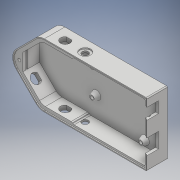
# Autodesk Inventor part: Arduino simple 4 channel ttl bottom
Saved by Autodesk Inventor 2017 (Build 210142000, 142)
## iProperties
Created: 2016-10-03
Part Number: Arduino simple 4 channel ttl bottom
Material: Generic
Document SubType Name: Modeling
Designer: andrew
Density: 1 g/cm^3
Appearance: Default
Author: andrew
Autodesk Inventor part; units mm, degrees
ref_plane "YZ Plane" through (0, 0, 0) normal (1, 0, 0) x (0, 1, 0)
ref_plane "XZ Plane" through (0, 0, 0) normal (0, 1, 0) x (-1, 0, 0)
ref_plane "XY Plane" through (0, 0, 0) normal (0, 0, 1) x (1, 0, 0)
sketch "Sketch1" plane through (0, 0, 0) normal (0, 1, 0) x (-1, 0, 0)
  circle A0 centre (66.1, -35.5) radius 2.345
  circle A1 centre (15.3, -50.7) radius 2.345
  circle A2 centre (14, -2.5) radius 2.345
  circle A3 centre (66.1, -7.6) radius 2.345
  line L0 (0, 0) -> (68.6, 0) construction
  line L1 (0, -53.3) -> (0, 0) construction
  line L2 (66.1, -53.3) -> (0, -53.3) construction
  line L3 (66.1, -40.6) -> (66.1, -53.3) construction
  line L4 (68.6, -40.6) -> (66.1, -40.6) construction
  line L5 (68.6, 0) -> (68.6, -40.6) construction
  line L6 (0, -12.2) -> (0, -3.3) construction
  line L7 (-1.8, -3.3) -> (0, -3.3) construction
  line L8 (-1.8, -12.2) -> (-1.8, -3.3) construction
  line L9 (0, -12.2) -> (-1.8, -12.2) construction
  line L10 (-6.2, -43.5895) -> (-6.2, -31.5895) construction
  line L11 (0, -43.5895) -> (0, -31.5895) construction
  line L12 (-6.2, -31.5895) -> (0, -31.5895) construction
  line L13 (-6.2, -43.5895) -> (-6.2, -31.5895) construction
  line L14 (0, -43.5895) -> (-6.2, -43.5895) construction
  circle A4 centre (14, -2.5) radius 1.6
  circle A5 centre (15.3, -50.7) radius 1.6
  circle A6 centre (66.1, -35.5) radius 1.6
  circle A7 centre (66.1, -7.6) radius 1.6
  constraints: 30 end point, 8 centre point
extrude "Extrusion1" add sketch "Sketch1" along normal blind 4.69
draft "FaceDraft1" angle 25 pull direction (0, -1, 0) faces at (-68.4146, 3.1267, -7.9762) (-64.2253, 3.1267, -36.9087) (-16.3146, 3.1267, -2.8762) (-17.6146, 3.1267, -51.0762) fixed edges at (-63.755, 0, -7.6) (-63.755, 0, -35.5) (-11.655, 0, -2.5) (-12.955, 0, -50.7)
sketch "Sketch2" plane through (-66.1, 4.69, -7.6) normal (0, 1, 0) x (1, 0, 0)
  circle A0 centre (0.0002, 27.8999) radius 2.345 construction
  circle A1 centre (50.8002, 43.0999) radius 2.345 construction
  circle A2 centre (52.1002, -5.1001) radius 2.345 construction
  circle A3 centre (0.0002, -0.0001) radius 2.345 construction
  line L0 (66.1002, -7.6001) -> (-2.4998, -7.6001) construction
  line L1 (66.1002, 45.6999) -> (66.1002, -7.6001) construction
  line L2 (0.0002, 45.6999) -> (66.1002, 45.6999) construction
  line L3 (0.0002, 32.9999) -> (0.0002, 45.6999) construction
  line L4 (-2.4998, 32.9999) -> (0.0002, 32.9999) construction
  line L5 (-2.4998, -7.6001) -> (-2.4998, 32.9999) construction
  line L6 (66.1002, 4.5999) -> (66.1002, -4.3001) construction
  line L7 (67.9002, -4.3001) -> (66.1002, -4.3001) construction
  line L8 (66.1002, 4.5999) -> (67.9002, 4.5999) construction
  line L9 (72.3002, 35.9894) -> (72.3002, 23.9894) construction
  line L10 (66.1002, 35.9894) -> (66.1002, 23.9894) construction
  line L11 (72.3002, 23.9894) -> (66.1002, 23.9894) construction
  line L12 (72.3002, 35.9894) -> (72.3002, 23.9894) construction
  line L13 (66.1002, 35.9894) -> (72.3002, 35.9894) construction
  circle A4 centre (52.1002, -5.1001) radius 1.6 construction
  circle A5 centre (50.8002, 43.0999) radius 1.6 construction
  circle A6 centre (0.0002, 27.8999) radius 1.6 construction
  circle A7 centre (0.0002, -0.0001) radius 1.6 construction
  line L14 (-4.4998, -9.6001) -> (68.1002, -9.6001) construction
  line L15 (-1.9998, 47.6999) -> (-1.9998, 34.9999) construction
  line L16 (-1.9998, 34.9999) -> (-4.4998, 34.9999) construction
  line L17 (66.1002, 4.5999) -> (74.6809, 4.5999) construction
  line L18 (74.6809, 4.5999) -> (74.6809, -4.3001) construction
  line L19 (74.6809, -4.3001) -> (66.1002, -4.3001) construction
  line L20 (66.1002, -4.3001) -> (66.1002, 4.5999) construction
  line L21 (66.1002, 23.9894) -> (80.0982, 23.9894) construction
  line L22 (80.0982, 23.9894) -> (80.0982, 35.9894) construction
  line L23 (80.0982, 35.9894) -> (66.1002, 35.9894) construction
  line L24 (66.1002, 35.9894) -> (66.1002, 23.9894) construction
  line L25 (76.0853, 6.0043) -> (64.6958, 6.0043) construction
  line L26 (64.6958, 6.0043) -> (64.6958, -5.7045) construction
  line L27 (64.6958, -5.7045) -> (76.0853, -5.7045) construction
  line L28 (76.0853, -5.7045) -> (76.0853, 6.0043) construction
  line L29 (82.0982, 21.9894) -> (64.1002, 21.9894) construction
  line L30 (64.1002, 21.9894) -> (64.1002, 37.9894) construction
  line L31 (64.1002, 37.9894) -> (82.0982, 37.9894) construction
  line L32 (82.0982, 37.9894) -> (82.0982, 21.9894) construction
  line L33 (68.1002, 6.0043) -> (71.1002, 6.0043)
  line L34 (71.1002, 21.9894) -> (68.1002, 21.9894)
  line L35 (71.1002, 37.9894) -> (68.1002, 37.9894)
  line L36 (68.1002, -5.7045) -> (68.1002, -9.6001)
  line L37 (68.1002, -9.6001) -> (68.1002, -4.3001) construction
  line L38 (68.1002, 6.0043) -> (68.1002, 47.6999) construction
  line L39 (68.1002, 47.6999) -> (68.1002, 37.9894)
  line L40 (68.1002, 21.9894) -> (68.1002, 6.0043)
  line L41 (71.1002, 37.9894) -> (71.1002, 50.6999)
  line L42 (68.1002, -9.6001) -> (68.1002, -11.1001)
  line L43 (68.1002, 47.6999) -> (68.1002, 49.1999)
  line L44 (68.1002, 47.6999) -> (69.6002, 47.6999) construction
  line L45 (71.1002, 50.6999) -> (71.1002, 52.1999)
  line L46 (71.1002, 50.6999) -> (72.6002, 50.6999) construction
  line L47 (68.1002, 49.1999) -> (-6.7498, 49.1999)
  line L48 (68.1002, -11.1001) -> (-6.7498, -11.1001)
  line L49 (71.1002, -14.1001) -> (71.1002, -5.7045)
  line L50 (71.1002, 6.0043) -> (71.1002, 21.9894)
  line L51 (71.1002, -5.7045) -> (68.1002, -5.7045)
  line L52 (-15.2028, 65.0749) -> (-15.2028, 33.3249) construction
  line L53 (-16.7928, 49.1999) -> (-16.7928, 33.3249) construction
  line L54 (-21.7478, 49.1999) -> (-16.7928, 49.1999) construction
  line L55 (-21.7478, 33.3249) -> (-21.7478, 65.0749) construction
  line L56 (-15.2028, 33.3249) -> (-28.2928, 33.3249) construction
  line L57 (-15.2028, 49.1999) -> (-28.2928, 49.1999) construction
  line L58 (-35.9958, 47.6999) -> (-8.2498, 47.6999)
  line L59 (-16.7928, 33.3249) -> (-26.7028, 33.3249) construction
  line L60 (-53.1418, 1.9038) -> (-56.6456, 5.4076) construction
  line L61 (-56.6456, 5.4076) -> (-45.4202, 16.6329) construction
  line L62 (-45.4202, 16.6329) -> (-38.4128, 9.6254) construction
  line L63 (-46.5445, 17.7572) -> (-37.2885, 8.5011) construction
  line L64 (-68.9952, -4.6935) -> (-46.5445, 17.7572) construction
  line L65 (-57.7699, 6.5319) -> (-48.5138, -2.7242) construction
  line L66 (-38.4128, 9.6254) -> (-49.6381, -1.5999) construction
  line L67 (-42.0062, -7.1105) -> (-62.1562, 13.0395)
  line L68 (-41.9165, 13.1292) -> (-64.3672, -9.3215) construction
  line L69 (-45.1882, -10.2925) -> (-65.3382, 9.8575)
  line L70 (-37.2885, 8.5011) -> (-59.7391, -13.9495) construction
  line L71 (-59.7391, -13.9495) -> (-68.9952, -4.6935) construction
  arc A8 (-65.3382, 28.2423) -> (-65.3382, 9.8575) centre (-56.1458, 19.0499) ccw
  arc A9 (-62.1562, 25.0603) -> (-62.1562, 13.0395) centre (-56.1458, 19.0499) ccw
  line L72 (-8.2498, -9.6001) -> (-35.9958, -9.6001)
  arc A10 (-42.0062, -7.1105) -> (-35.9958, -9.6001) centre (-35.9958, -1.1001) ccw
  arc A11 (-45.1882, -10.2925) -> (-35.9958, -14.1001) centre (-35.9958, -1.1001) ccw
  line L73 (-28.2928, 33.3249) -> (-28.2928, 65.0749) construction
  line L74 (-26.7028, 33.3249) -> (-26.7028, 49.1999) construction
  arc A12 (-35.9958, 47.6999) -> (-42.0062, 45.2103) centre (-35.9958, 39.1999) ccw
  arc A13 (-35.9958, 52.1999) -> (-45.1882, 48.3923) centre (-35.9958, 39.1999) ccw
  line L75 (-65.3382, 28.2423) -> (-45.1882, 48.3923)
  line L76 (-62.1562, 25.0603) -> (-42.0062, 45.2103)
  line L77 (-7.4998, -10.3501) -> (-7.4998, -10.3501)
  line L78 (-7.4998, 48.4499) -> (-7.4998, 48.4499)
  line L79 (-35.9958, -14.1001) -> (71.1002, -14.1001)
  line L80 (-35.9958, 52.1999) -> (71.1002, 52.1999)
  line L81 (-8.2498, -9.6001) -> (-6.7498, -11.1001)
  line L82 (-8.2498, 47.6999) -> (-6.7498, 49.1999)
  line L83 (-52.0812, 2.9645) -> (-59.329, 10.2123) construction
  line L84 (-59.329, 10.2123) -> (-59.329, 27.8875) construction
  point P0 (66.1, -7.6)
  point P1 (66.1002, -7.6001)
  point P2 (-40.1379, -11.1001)
  point P3 (-70.2879, 19.0499)
  dimension "d7" = 2
  dimension "d9" = 2
  dimension "d51" = 1.5
  dimension "d53" = 1.5
  dimension "d54" = 90
  dimension "d55" = 1.5
  dimension "d56" = 90
  dimension "d146" = 4.955
  dimension "d147" = 9.91
  dimension "d152" = 31.75
  dimension "d153" = 13.09
  dimension "d154" = 4.955
  dimension "d155" = 9.91
  dimension "d204" = 10.25
  dimension "d205" = 17.6751
  constraints: 170 end point, 20 point on line, 14 centre point, 13 perpendicular, 12 point on circle, 11 parallel, 10 midpoint, 8 horizontal, 5 vertical, 1 coincident, 1 collinear, 11 other
  measures "d7" distance between parallel lines of L0 L14
  measures "d9" distance between parallel lines of L21 L29
  measures "d51" distance of L14.end L42.end
  measures "d53" distance of L38.end L43.end
  measures "d54" angle of L44 L43
  measures "d55" distance of L41.end L45.end
  measures "d56" angle of L46 L45
  measures "d146" distance of L60.start L60.end
  measures "d147" distance of L62.start L66.start
  measures "d152" distance of L56.end L73.end
  measures "d153" distance of L56.start L56.end
  measures "d154" distance of L54.start L53.start
  measures "d155" distance of L59.start L74.start
  measures "d204" distance of L83.start L83.end
  measures "d205" distance of L83.end L84.end
extrude "Extrusion2" add sketch "Sketch2" against normal blind 17.29
sketch "Sketch4" plane through (-66.1, -12.6, -7.6) normal (0, -1, 0) x (1, 0, 0)
  line L0 (-85.6267, 83.4161) -> (-53.8767, 83.4161)
  line L1 (-53.8767, 83.4161) -> (-53.8767, 70.3261)
  line L2 (-53.8767, 70.3261) -> (-85.6267, 70.3261)
  line L3 (-85.6267, 70.3261) -> (-85.6267, 83.4161)
  line L4 (-53.8767, 76.8711) -> (-85.6267, 76.8711)
  line L5 (-69.7517, 83.4161) -> (-69.7517, 70.3261)
  line L6 (-69.7517, 76.8711) -> (-69.7517, 81.8261)
  line L7 (-69.7517, 81.8261) -> (-53.8767, 81.8261)
  line L8 (-53.8767, 81.8261) -> (-53.8767, 71.9161)
  line L9 (-53.8767, 71.9161) -> (-69.7517, 71.9161)
  line L10 (-85.7515, 30.5625) -> (-63.3008, 53.0132)
  line L11 (-63.3008, 53.0132) -> (-54.0448, 43.7571)
  line L12 (-54.0448, 43.7571) -> (-76.4954, 21.3065)
  line L13 (-76.4954, 21.3065) -> (-85.7515, 30.5625)
  line L14 (-58.6728, 48.3851) -> (-81.1234, 25.9345)
  line L15 (-74.5261, 41.7878) -> (-65.2701, 32.5318)
  line L16 (-69.8981, 37.1598) -> (-73.4018, 40.6635)
  line L17 (-73.4018, 40.6635) -> (-62.1765, 51.8889)
  line L18 (-62.1765, 51.8889) -> (-55.1691, 44.8814)
  line L19 (-55.1691, 44.8814) -> (-66.3944, 33.6561)
  line L20 (-56.2658, 116.7338) -> (-33.8151, 94.2832)
  line L21 (-33.8151, 94.2832) -> (-43.0711, 85.0271)
  line L22 (-43.0711, 85.0271) -> (-65.5218, 107.4778)
  line L23 (-65.5218, 107.4778) -> (-56.2658, 116.7338)
  line L24 (-38.4431, 89.6551) -> (-60.8938, 112.1058)
  line L25 (-45.0404, 105.5085) -> (-54.2965, 96.2524)
  line L26 (-49.6685, 100.8805) -> (-46.1647, 104.3842)
  line L27 (-46.1647, 104.3842) -> (-34.9394, 93.1589)
  line L28 (-34.9394, 93.1589) -> (-41.9468, 86.1514)
  line L29 (-41.9468, 86.1514) -> (-53.1722, 97.3767)
  line L30 (71.1002, -52.1999) -> (-7.4998, -52.1999)
  line L31 (-7.4998, -52.1999) -> (-7.4998, 14.1001)
  line L32 (-7.4998, 14.1001) -> (71.1002, 14.1001)
  line L33 (71.1002, 14.1001) -> (71.1002, -52.1999)
  line L34 (68.1002, 11.1001) -> (68.1002, 5.7045) projected
  line L35 (68.1002, -49.1999) -> (-6.7498, -49.1999) projected
  line L36 (68.1002, 11.1001) -> (-4.4998, 11.1001)
  line L37 (-4.4998, 11.1001) -> (-4.4998, -49.1999)
  line L38 (-4.4998, -49.1999) -> (68.1002, -49.1999)
  line L39 (68.1002, -49.1999) -> (68.1002, 11.1001)
  line L40 (-4.4998, -49.1999) -> (34.0716, -49.1999) construction
  line L41 (-7.4998, 14.1001) -> (-7.4998, -52.1999) projected
  line L42 (-7.4998, -19.0499) -> (35.1392, -19.0499) construction
  line L43 (-38.4431, -92.3206) -> (-68.5931, -122.4706)
  line L44 (-38.4431, -152.6206) -> (-68.5931, -122.4706)
  line L45 (-69.3715, -144.1429) -> (-46.9208, -121.6922)
  line L46 (-46.9208, -121.6922) -> (-37.6648, -130.9483)
  line L47 (-37.6648, -130.9483) -> (-60.1154, -153.3989)
  line L48 (-38.7891, -129.824) -> (-50.0144, -141.0493)
  line L49 (-45.7965, -122.8165) -> (-38.7891, -129.824)
  line L50 (-57.0218, -134.0419) -> (-45.7965, -122.8165)
  line L51 (-53.5181, -137.5456) -> (-57.0218, -134.0419)
  line L52 (-58.1461, -132.9176) -> (-48.8901, -142.1736)
  line L53 (-60.1154, -153.3989) -> (-69.3715, -144.1429)
  line L54 (-42.2928, -126.3203) -> (-64.7435, -148.7709)
  line L55 (-37.6648, -113.9929) -> (-46.9208, -123.2489)
  line L56 (-38.7891, -115.1172) -> (-45.7965, -122.1246)
  line L57 (-45.7965, -122.1246) -> (-57.0218, -110.8993)
  line L58 (-50.0144, -103.8919) -> (-38.7891, -115.1172)
  line L59 (-48.8901, -102.7676) -> (-58.1461, -112.0236)
  line L60 (-46.9208, -123.2489) -> (-69.3715, -100.7983)
  line L61 (-42.2928, -118.6209) -> (-64.7435, -96.1703)
  line L62 (-60.1154, -91.5422) -> (-37.6648, -113.9929)
  line L63 (-69.3715, -100.7983) -> (-60.1154, -91.5422)
  line L64 (-53.5181, -107.3956) -> (-50.0144, -103.8919)
  line L65 (58.0279, 196.0229) -> (58.0279, 164.2729)
  line L66 (58.0279, 164.2729) -> (44.9379, 164.2729)
  line L67 (44.9379, 164.2729) -> (44.9379, 196.0229)
  line L68 (44.9379, 196.0229) -> (58.0279, 196.0229)
  line L69 (51.4829, 164.2729) -> (51.4829, 196.0229)
  line L70 (58.0279, 180.1479) -> (44.9379, 180.1479)
  line L71 (51.4829, 180.1479) -> (56.4379, 180.1479)
  line L72 (56.4379, 180.1479) -> (56.4379, 164.2729)
  line L73 (56.4379, 164.2729) -> (46.5279, 164.2729)
  line L74 (46.5279, 164.2729) -> (46.5279, 180.1479)
  line L75 (-7.4998, 14.1001) -> (-7.4998, -52.1999)
  line L76 (-68.9952, -42.7933) -> (-46.5445, -20.3426) construction
  line L77 (-46.5445, -20.3426) -> (-37.2885, -29.5987) construction
  line L78 (-37.2885, -29.5987) -> (-59.7391, -52.0493) construction
  line L79 (-38.4128, -28.4744) -> (-49.6381, -39.6997) construction
  line L80 (-41.9165, -24.9707) -> (-64.3672, -47.4213) construction
  line L81 (-59.7391, -52.0493) -> (-68.9952, -42.7933)
  line L82 (-53.1418, -36.196) -> (-56.6456, -32.6923) construction
  line L83 (-57.7699, -31.568) -> (-48.5138, -40.824) construction
  line L84 (-45.4202, -21.4669) -> (-38.4128, -28.4744) construction
  line L85 (-56.6456, -32.6923) -> (-45.4202, -21.4669) construction
  line L86 (-58.8047, 14.9002) -> (-36.3541, -7.5505) construction
  line L87 (-36.3541, -7.5505) -> (-45.6101, -16.8065) construction
  line L88 (-45.6101, -16.8065) -> (-68.0607, 5.6441) construction
  line L89 (-68.0607, 5.6441) -> (-58.8047, 14.9002)
  line L90 (-40.9821, -12.1785) -> (-63.4327, 10.2722) construction
  line L91 (-44.4858, -15.6822) -> (-55.7111, -4.4569) construction
  line L92 (-52.2074, -0.9532) -> (-48.7037, 2.5506)
  line L93 (-48.7037, 2.5506) -> (-37.4784, -8.6748) construction
  line L94 (-37.4784, -8.6748) -> (-44.4858, -15.6822) construction
  line L95 (-47.5794, 3.6749) -> (-56.8354, -5.5812) construction
  line L96 (-15.2028, 26.9751) -> (-15.2028, -4.7749) construction
  line L97 (-15.2028, -4.7749) -> (-28.2928, -4.7749) construction
  line L98 (-28.2928, -4.7749) -> (-28.2928, 26.9751) construction
  line L99 (-28.2928, 26.9751) -> (-15.2028, 26.9751) construction
  line L100 (-21.7478, -4.7749) -> (-21.7478, 26.9751) construction
  line L101 (-16.7928, 11.1001) -> (-16.7928, -4.7749) construction
  line L102 (-21.7478, 11.1001) -> (-16.7928, 11.1001) construction
  line L103 (-16.7928, -4.7749) -> (-26.7028, -4.7749) construction
  line L104 (-26.7028, -4.7749) -> (-26.7028, 11.1001) construction
  line L105 (-15.2028, 11.1001) -> (-28.2928, 11.1001) construction
  line L106 (-4.4998, 11.1001) -> (-7.4998, 11.1001)
  line L107 (-7.4998, -52.1999) -> (-35.9958, -52.1999)
  arc A0 (-45.1882, -48.3923) -> (-35.9958, -52.1999) centre (-35.9958, -39.1999) ccw
  line L108 (-45.1882, -48.3923) -> (-65.3382, -28.2423)
  arc A1 (-65.3382, -9.8575) -> (-65.3382, -28.2423) centre (-56.1458, -19.0499) ccw
  line L109 (-65.3382, -9.8575) -> (-45.1882, 10.2925)
  arc A2 (-35.9958, 14.1001) -> (-45.1882, 10.2925) centre (-35.9958, 1.1001) ccw
  line L110 (-35.9958, 14.1001) -> (-7.4998, 14.1001)
  line L111 (-7.4998, -47.6999) -> (-35.9958, -47.6999)
  arc A3 (-42.0062, -45.2103) -> (-35.9958, -47.6999) centre (-35.9958, -39.1999) ccw
  line L112 (-42.0062, -45.2103) -> (-62.1562, -25.0603)
  arc A4 (-62.1562, -13.0395) -> (-62.1562, -25.0603) centre (-56.1458, -19.0499) ccw
  line L113 (-62.1562, -13.0395) -> (-42.0062, 7.1105)
  arc A5 (-35.9958, 9.6001) -> (-42.0062, 7.1105) centre (-35.9958, 1.1001) ccw
  line L114 (-35.9958, 9.6001) -> (-7.4998, 9.6001)
  point P0 (-70.2879, -19.0499)
  point P1 (-40.1379, -49.1999)
  dimension "d12" = 31.75
  dimension "d13" = 13.09
  dimension "d14" = 4.955
  dimension "d15" = 9.91
  dimension "d34" = 13.09
  dimension "d35" = 4.955
  dimension "d36" = 9.91
  dimension "d42" = 31.75
  dimension "d43" = 13.09
  dimension "d44" = 4.955
  dimension "d45" = 9.91
  dimension "d77" = 13.09
  dimension "d78" = 4.955
  dimension "d79" = 9.91
  dimension "d80" = 31.75
  dimension "d81" = 13.09
  dimension "d82" = 4.955
  dimension "d83" = 9.91
  dimension "d84" = 42.6385
  dimension "d92" = 42.6385
  dimension "d93" = 31.75
  dimension "d94" = 13.09
  dimension "d95" = 4.955
  dimension "d96" = 9.91
  dimension "d102" = 13.09
  dimension "d103" = 4.955
  dimension "d104" = 9.91
  dimension "d105" = 31.75
  dimension "d106" = 13.09
  dimension "d107" = 4.955
  dimension "d108" = 9.91
  dimension "d111" = 31.75
  dimension "d112" = 13.09
  dimension "d113" = 4.955
  dimension "d114" = 9.91
  dimension "d117" = 4.5
  constraints: 224 end point, 46 midpoint, 37 point on line, 30 perpendicular, 23 equal length, 12 point on circle, 6 centre point, 5 horizontal, 6 other
  measures "d12" distance of L1.end L2.end
  measures "d13" distance of L0.end L1.end
  measures "d14" distance of L6.start L6.end
  measures "d15" distance of L7.end L8.end
  measures "d34" distance of L10.end L11.end
  measures "d35" distance of L16.start L16.end
  measures "d36" distance of L18.start L19.start
  measures "d42" distance of L21.end L22.end
  measures "d43" distance of L20.end L21.end
  measures "d44" distance of L26.start L26.end
  measures "d45" distance of L27.end L29.start
  measures "d77" distance of L46.start L46.end
  measures "d78" distance of L51.start L50.start
  measures "d79" distance of L49.start L48.start
  measures "d80" distance of L55.end L63.start
  measures "d81" distance of L62.end L55.end
  measures "d82" distance of L64.start L64.end
  measures "d83" distance of L58.end L56.end
  measures "d84" distance of L44.start L43.end
  measures "d92" distance of point (-40.138, -49.2) point (-70.288, -19.05)
  measures "d93" distance of L66.end L67.end
  measures "d94" distance of L65.end L66.end
  measures "d95" distance of L71.start L72.start
  measures "d96" distance of L72.end L73.end
  measures "d102" distance of L77.start L77.end
  measures "d103" distance of L82.start L85.start
  measures "d104" distance of L84.start L84.end
  measures "d105" distance of L87.end L89.start
  measures "d106" distance of L87.start L87.end
  measures "d107" distance of L92.start L92.end
  measures "d108" distance of L94.start L91.start
  measures "d111" distance of L97.end L98.end
  measures "d112" distance of L96.end L97.end
  measures "d113" distance of L102.start L101.start
  measures "d114" distance of L103.start L103.end
  measures "d117" radial gap between concentric circles of A2 A5
fillet "Fillet1" radius 2 4 edges at (-74.3498, -3.955, -55.2999) (-72.8498, -3.955, -56.7999) (-74.3498, -3.955, 2.0001) (-72.8498, -3.955, 3.5001)
sketch "Sketch5" plane through (5.0002, 4.69, -59.7999) normal (0, 0, -1) x (-1, 0, 0)
  line L0 (80.1784, -17.29) -> (107.096, -17.29) construction
  line L1 (107.096, -17.29) -> (107.096, 0) construction
  line L2 (107.096, 0) -> (80.1784, 0) construction
  line L3 (80.1784, 0) -> (80.1784, -17.29) construction
  line L4 (107.096, 0) -> (107.096, -17.29) construction
  line L5 (107.096, -8.645) -> (80.1784, -8.645) construction
  line L6 (80.1784, 0) -> (80.1784, -17.29) construction
  arc A0 (91.5414, -5.11) -> (97.6798, -5.11) centre (94.6106, -9) ccw
  line L7 (91.5414, -5.11) -> (97.6798, -5.11)
  line L8 (86.3603, -8.645) -> (90.4854, -1.5) construction
  line L9 (90.4854, -1.5) -> (98.7358, -1.5) construction
  line L10 (98.7358, -1.5) -> (102.8609, -8.645) construction
  line L11 (102.8609, -8.645) -> (98.7358, -15.79) construction
  line L12 (98.7358, -15.79) -> (90.4854, -15.79) construction
  line L13 (90.4854, -15.79) -> (86.3603, -8.645) construction
  line L14 (94.6106, -8.645) -> (90.4854, -1.5) construction
  line L15 (94.6106, -9) -> (94.6106, -0.75) construction
  line L16 (0, 0) -> (107.096, 0) construction
  line L17 (94.6106, -8) -> (102.8606, -8) construction
  line L18 (94.6106, 0) -> (94.6106, 0.1979) construction
  line L19 (94.6106, -8) -> (94.6106, -9) construction
  line L20 (94.6106, -8) -> (95.6106, -8) construction
  point P0 (5.0002, -4.69)
  dimension "d160" = 9.91
  dimension "d180" = 14.29
  dimension "d181" = 8.2503
  dimension "d182" = 8.25
  dimension "d183" = 90
  dimension "d185" = 0.75
  dimension "d186" = 1
  dimension "d187" = 90
  dimension "d199" = 6.1818
  constraints: 36 end point, 4 horizontal, 4 perpendicular, 2 midpoint, 2 parallel, 2 point on circle, 2 point on line, 1 centre point, 1 coincident, 1 vertical, 1 other
  measures "d160" diameter of A0
  measures "d180" distance between parallel lines of L9 L12
  measures "d181" distance of L14.start L8.end
  measures "d182" distance of L15.start L15.end
  measures "d183" angle of L17 L15
  measures "d185" distance of L15.end L18.start
  measures "d186" distance of L19.start L19.end
  measures "d187" angle of L19 L20
  measures "d199" distance from line of L3 L8.start
extrude "Extrusion3" cut sketch "Sketch5" against normal blind 100
sketch "Sketch6" plane through (-111.2882, -12.6, -55.9923) normal (-0.7071068, 0, -0.7071068) x (-0.7071068, 0, 0.7071068)
  arc A0 (12.3053, 10.8312) -> (18.6412, 10.8312) centre (15.4732, 7.0212) ccw
  line L0 (15.4732, 7.0212) -> (15.4732, 10.8312)
  line L1 (12.3053, 10.8312) -> (18.6412, 10.8312)
  line L2 (15.4732, 8.0212) -> (15.4732, 7.0212)
  line L3 (15.4732, 0) -> (15.4732, 17.29) projected
  line L4 (15.4732, 8.0212) -> (16.4732, 8.0212) construction
  point P0 (-39.1001, 12.6)
  point P1 (28.4964, 16)
  dimension "d164" = 9.91
  dimension "d165" = 3.81
  dimension "d188" = 1
  dimension "d189" = 90
  constraints: 8 end point, 2 horizontal, 2 point on circle, 1 centre point, 1 collinear, 1 perpendicular
  measures "d164" diameter of A0
  measures "d165" distance of L0.start L0.end
  measures "d188" distance of L2.start L2.end
  measures "d189" angle of L2 L4
extrude "Extrusion4" cut sketch "Sketch6" against normal blind 10
sketch "Sketch7" plane through (-131.4382, -12.6, -17.4575) normal (-0.7071068, 0, 0.7071068) x (0.7071068, 0, 0.7071068)
  line L0 (28.4964, 8) -> (0, 8) construction
  line L1 (14.1948, 7) -> (14.1948, 0) construction
  arc A0 (11.1256, 10.89) -> (17.264, 10.89) centre (14.1948, 7) ccw
  line L2 (14.1948, 0) -> (14.1948, 17.29) projected
  line L3 (14.1948, 8) -> (18.0848, 8) construction
  line L4 (11.1256, 10.89) -> (17.264, 10.89)
  line L5 (14.1948, 14.245) -> (14.1948, 17.29)
  line L6 (21.1672, 8) -> (21.1672, 7)
  line L7 (21.1672, 8) -> (22.1672, 8) construction
  point P0 (105.2851, 12.6)
  dimension "d171" = 9.91
  dimension "d179" = 3.045
  dimension "d190" = 1
  dimension "d191" = 90
  constraints: 14 end point, 2 horizontal, 2 point on circle, 2 point on line, 1 centre point, 1 coincident, 1 collinear, 1 perpendicular, 1 vertical
  measures "d171" diameter of A0
  measures "d179" distance of L2.end L5.start
  measures "d190" distance of L6.start L6.end
  measures "d191" angle of L6 L7
extrude "Extrusion5" cut sketch "Sketch7" against normal blind 10
fillet "Fillet2" radius 1 4 edges at (2.0002, -3.955, -56.7999) (2.0002, -3.955, 3.5001) (5.0002, -3.955, -59.7999) (5.0002, -3.955, 6.5001)
sketch "Sketch8" plane through (-66.1, 4.69, -7.6) normal (0, 1, 0) x (1, 0, 0)
  arc A0 (70.1002, -14.1001) -> (71.1002, -13.1001) centre (70.1002, -13.1001) ccw projected
  line L0 (71.1002, -5.7045) -> (71.1002, -13.1001) projected
  line L1 (68.1002, -5.7045) -> (71.1002, -5.7045) projected
  line L2 (68.1002, -10.1001) -> (68.1002, -5.7045) projected
  arc A1 (67.1002, -11.1001) -> (68.1002, -10.1001) centre (67.1002, -10.1001) ccw projected
  line L3 (-5.9213, -11.1001) -> (67.1002, -11.1001) projected
  arc A2 (-7.3356, -10.5143) -> (-5.9213, -11.1001) centre (-5.9213, -9.1001) ccw projected
  line L4 (-7.664, -10.1859) -> (-7.3356, -10.5143) projected
  arc A3 (-7.664, -10.1859) -> (-9.0782, -9.6001) centre (-9.0782, -11.6001) ccw projected
  line L5 (-35.9958, -9.6001) -> (-9.0782, -9.6001) projected
  arc A4 (-42.0062, -7.1105) -> (-35.9958, -9.6001) centre (-35.9958, -1.1001) ccw projected
  line L6 (-62.1562, 13.0395) -> (-42.0062, -7.1105) projected
  arc A5 (-62.1562, 25.0603) -> (-62.1562, 13.0395) centre (-56.1458, 19.0499) ccw projected
  line L7 (-42.0062, 45.2103) -> (-62.1562, 25.0603) projected
  arc A6 (-35.9958, 47.6999) -> (-42.0062, 45.2103) centre (-35.9958, 39.1999) ccw projected
  line L8 (-9.0782, 47.6999) -> (-35.9958, 47.6999) projected
  arc A7 (-9.0782, 47.6999) -> (-7.664, 48.2857) centre (-9.0782, 49.6999) ccw projected
  line L9 (-7.3356, 48.6141) -> (-7.664, 48.2857) projected
  arc A8 (-5.9213, 49.1999) -> (-7.3356, 48.6141) centre (-5.9213, 47.1999) ccw projected
  line L10 (67.1002, 49.1999) -> (-5.9213, 49.1999) projected
  arc A9 (68.1002, 48.1999) -> (67.1002, 49.1999) centre (67.1002, 48.1999) ccw projected
  line L11 (68.1002, 37.9894) -> (68.1002, 48.1999) projected
  line L12 (71.1002, 37.9894) -> (68.1002, 37.9894) projected
  line L13 (71.1002, 51.1999) -> (71.1002, 37.9894) projected
  arc A10 (71.1002, 51.1999) -> (70.1002, 52.1999) centre (70.1002, 51.1999) ccw projected
  line L14 (-35.9958, 52.1999) -> (70.1002, 52.1999) projected
  arc A11 (-35.9958, 52.1999) -> (-45.1882, 48.3923) centre (-35.9958, 39.1999) ccw projected
  line L15 (-65.3382, 28.2423) -> (-45.1882, 48.3923) projected
  arc A12 (-65.3382, 28.2423) -> (-65.3382, 9.8575) centre (-56.1458, 19.0499) ccw projected
  line L16 (-45.1882, -10.2925) -> (-65.3382, 9.8575) projected
  arc A13 (-45.1882, -10.2925) -> (-35.9958, -14.1001) centre (-35.9958, -1.1001) ccw projected
  line L17 (70.1002, -14.1001) -> (-35.9958, -14.1001) projected
  line L18 (71.1002, 37.9894) -> (71.1002, -5.7045)
  constraints: 2 end point, 1 vertical
extrude "Extrusion6" add sketch "Sketch8" along normal blind 3
sketch "Sketch9" plane through (-66.1, 4.69, -7.6) normal (0, -1, 0) x (1, 0, 0)
  line L0 (68.1002, 10.1001) -> (68.1002, 5.7045) projected
  line L1 (71.1002, -37.9894) -> (68.1002, -37.9894) projected
  line L2 (68.1002, 5.7045) -> (71.1002, 5.7045)
  line L3 (71.1002, 5.7045) -> (71.1002, -37.9894)
  line L4 (71.1002, -37.9894) -> (68.1002, -37.9894)
  line L5 (68.1002, -37.9894) -> (68.1002, 5.7045)
  point P0 (66.1, 7.6)
  constraints: 8 end point, 2 parallel, 1 horizontal, 1 perpendicular
extrude "Extrusion7" add sketch "Sketch9" along normal blind 6.29
sketch "Sketch10" plane through (-66.1, -12.6, -7.6) normal (0, -1, 0) x (1, 0, 0)
  arc A0 (71.1002, 13.1001) -> (70.1002, 14.1001) centre (70.1002, 13.1001) ccw projected
  line L0 (70.1002, 14.1001) -> (-35.9958, 14.1001) projected
  arc A1 (-35.9958, 14.1001) -> (-45.1882, 10.2925) centre (-35.9958, 1.1001) ccw projected
  line L1 (-45.1882, 10.2925) -> (-65.3382, -9.8575) projected
  arc A2 (-65.3382, -9.8575) -> (-65.3382, -28.2423) centre (-56.1458, -19.0499) ccw projected
  line L2 (-65.3382, -28.2423) -> (-45.1882, -48.3923) projected
  arc A3 (-45.1882, -48.3923) -> (-35.9958, -52.1999) centre (-35.9958, -39.1999) ccw projected
  line L3 (-35.9958, -52.1999) -> (70.1002, -52.1999) projected
  arc A4 (70.1002, -52.1999) -> (71.1002, -51.1999) centre (70.1002, -51.1999) ccw projected
  line L4 (71.1002, -51.1999) -> (71.1002, -37.9894) projected
  line L5 (71.1002, -37.9894) -> (68.1002, -37.9894) projected
  line L6 (68.1002, -37.9894) -> (68.1002, -48.1999) projected
  arc A5 (67.1002, -49.1999) -> (68.1002, -48.1999) centre (67.1002, -48.1999) ccw projected
  line L7 (67.1002, -49.1999) -> (-5.9213, -49.1999) projected
  arc A6 (-7.3356, -48.6141) -> (-5.9213, -49.1999) centre (-5.9213, -47.1999) ccw projected
  line L8 (-7.3356, -48.6141) -> (-7.664, -48.2857) projected
  arc A7 (-7.664, -48.2857) -> (-9.0782, -47.6999) centre (-9.0782, -49.6999) ccw projected
  line L9 (-9.0782, -47.6999) -> (-35.9958, -47.6999) projected
  arc A8 (-42.0062, -45.2103) -> (-35.9958, -47.6999) centre (-35.9958, -39.1999) ccw projected
  line L10 (-42.0062, -45.2103) -> (-62.1562, -25.0603) projected
  arc A9 (-62.1562, -13.0395) -> (-62.1562, -25.0603) centre (-56.1458, -19.0499) ccw projected
  line L11 (-62.1562, -13.0395) -> (-42.0062, 7.1105) projected
  arc A10 (-35.9958, 9.6001) -> (-42.0062, 7.1105) centre (-35.9958, 1.1001) ccw projected
  line L12 (-35.9958, 9.6001) -> (-9.0782, 9.6001) projected
  arc A11 (-9.0782, 9.6001) -> (-7.664, 10.1859) centre (-9.0782, 11.6001) ccw projected
  line L13 (-7.664, 10.1859) -> (-7.3356, 10.5143) projected
  arc A12 (-5.9213, 11.1001) -> (-7.3356, 10.5143) centre (-5.9213, 9.1001) ccw projected
  line L14 (-5.9213, 11.1001) -> (67.1002, 11.1001) projected
  arc A13 (68.1002, 10.1001) -> (67.1002, 11.1001) centre (67.1002, 10.1001) ccw projected
  line L15 (68.1002, 10.1001) -> (68.1002, 5.7045) projected
  line L16 (68.1002, 5.7045) -> (71.1002, 5.7045) projected
  line L17 (71.1002, 5.7045) -> (71.1002, 13.1001) projected
  line L18 (68.1002, -21.9894) -> (71.1002, -21.9894) projected
  line L19 (71.1002, -21.9894) -> (71.1002, -6.0043) projected
  line L20 (71.1002, -6.0043) -> (68.1002, -6.0043) projected
  line L21 (68.1002, -6.0043) -> (68.1002, -21.9894) projected
  line L22 (-35.9958, 13.1001) -> (70.1002, 13.1001)
  line L23 (70.1002, 13.1001) -> (70.1002, 5.7045)
  line L24 (70.1002, -51.1999) -> (-35.9958, -51.1999)
  arc A14 (-44.4811, -47.6852) -> (-35.9958, -51.1999) centre (-35.9958, -39.1999) ccw
  line L25 (-44.4811, -47.6852) -> (-64.6311, -27.5352)
  arc A15 (-64.6311, -10.5646) -> (-64.6311, -27.5352) centre (-56.1458, -19.0499) ccw
  line L26 (-64.6311, -10.5646) -> (-44.4811, 9.5854)
  arc A16 (-35.9958, 13.1001) -> (-44.4811, 9.5854) centre (-35.9958, 1.1001) ccw
  line L27 (70.1002, -6.0043) -> (70.1002, -21.9894)
  line L28 (70.1002, -37.9894) -> (70.1002, -51.1999)
  point P0 (66.1, 7.6)
  dimension "d194" = 1
  constraints: 14 end point, 6 point on circle, 4 point on line, 3 centre point, 5 other
  measures "d194" distance between parallel lines of L0 L22
extrude "Extrusion8" add sketch "Sketch10" along normal blind 1 contours L17 L16 L23 L22 A16 L26 A15 L25 A14 L24 L28 L5 L4 A4 L3 A3 L2 A2 L1 A1 L0 A0 | L27 L20 L19 L18
sketch "Sketch13" plane through (-66.1, -12.6, -7.6) normal (0, -1, 0) x (1, 0, 0)
  line L0 (-59.329, -10.2123) -> (-59.329, -27.8875)
  line L1 (-59.329, -10.2123) -> (-60.2707, -9.2706)
  line L2 (-60.2707, -9.2706) -> (-65.5374, -14.5373)
  line L3 (-65.5374, -14.5373) -> (-65.5374, -23.7339)
  line L4 (-65.5374, -23.7339) -> (-59.329, -29.9423)
  line L5 (-59.329, -29.9423) -> (-59.329, -27.8875)
  line L6 (-59.329, -19.0499) -> (-80.366, -19.0499) construction
  circle A0 centre (-63.0458, -19.0499) radius 1.6
  arc A1 (-62.1562, -13.0395) -> (-62.1562, -25.0603) centre (-56.1458, -19.0499) ccw construction
  line L7 (-64.6458, -19.0499) -> (-76.6779, -19.0499) construction
  line L8 (-82.9257, -9.0889) -> (-87.7423, -9.0889) construction
  line L9 (-84.5257, -9.0889) -> (-86.6689, -9.0889) construction
  arc A2 (-65.3382, -9.8575) -> (-65.3382, -28.2423) centre (-56.1458, -19.0499) ccw projected
  dimension "d209" = 3.2
  constraints: 20 end point, 5 point on line, 2 horizontal, 2 parallel, 2 vertical, 1 centre point, 1 midpoint, 1 perpendicular, 1 point on circle
  measures "d209" diameter of A0
extrude "Extrusion9" add sketch "Sketch13" against normal blind 20
sketch "Sketch14" plane through (2.0002, -12.6, -29.5894) normal (-1, 0, 0) x (0, 0, 1)
  line L0 (15.9851, 11) -> (15.9851, -1) construction
  line L1 (0, 11) -> (0, -1) construction
  line L2 (0, 0) -> (15.9851, 0) construction
  line L3 (7.9925, 0) -> (7.9925, 3) construction
  line L4 (7.9925, 3) -> (15.9851, 3) construction
  line L5 (15.9851, 3) -> (15.9851, 5) construction
  line L6 (15.9851, 11) -> (15.9851, 0) construction
  line L7 (15.9851, 5) -> (0, 5) construction
  line L8 (15.9851, 3) -> (0, 3)
  line L9 (0, 3) -> (0, 5)
  line L10 (0, 5) -> (15.9851, 5)
  line L11 (15.9851, 5) -> (15.9851, 3)
  point P0 (29.5894, 12.6)
  dimension "d210" = 3
  dimension "d211" = 2
  constraints: 16 end point, 2 midpoint, 2 parallel, 2 perpendicular, 2 point on line, 1 horizontal, 1 vertical
  measures "d210" distance of L3.start L3.end
  measures "d211" distance of L4.end L5.end
extrude "Extrusion10" cut sketch "Sketch14" against normal blind 1
sketch "Sketch15" plane through (-125.429, -12.6, -17.8123) normal (1, 0, 0) x (0, 0, -1)
  line L0 (17.6751, 17.29) -> (17.6751, 0) construction
  line L1 (0, 17.29) -> (17.6751, 17.29) construction
  line L2 (0, 0) -> (0, 17.29) construction
  line L3 (17.6751, 0) -> (0, 0) construction
  line L4 (8.8376, 0) -> (8.8376, 3) construction
  line L5 (8.8376, 0) -> (11.8376, 0) construction
  line L6 (8.8376, 3) -> (0, 3) construction
  line L7 (0, 3) -> (0, 5) construction
  line L8 (0, 0) -> (0, 17.29) construction
  line L9 (0, 5) -> (17.6751, 5) construction
  line L10 (17.6751, 17.29) -> (17.6751, 0) construction
  line L11 (0, 3) -> (17.6751, 3)
  line L12 (17.6751, 3) -> (17.6751, 5)
  line L13 (17.6751, 5) -> (0, 5)
  line L14 (0, 5) -> (0, 3)
  point P0 (-17.8123, 12.6)
  dimension "d214" = 3
  dimension "d215" = 90
  dimension "d216" = 2
  constraints: 18 end point, 4 perpendicular, 3 point on line, 2 horizontal, 2 parallel, 1 midpoint, 1 vertical
  measures "d214" distance of L4.start L4.end
  measures "d215" angle of L5 L4
  measures "d216" distance of L6.end L7.end
extrude "Extrusion11" cut sketch "Sketch15" against normal blind 1
sketch "Sketch17" plane through (-102.0958, 7.69, 6.5001) normal (0, 0, 1) x (1, 0, 0)
  arc A0 (9.4162, -8.11) -> (15.5546, -8.11) centre (12.4854, -12) ccw projected
  line L0 (30.0744, -20.29) -> (30.0744, -3) projected
  circle A1 centre (12.4854, -12) radius 17.5926
  circle A2 centre (33.328, -12) radius 3.25
  point P0 (102.0958, -7.69)
  dimension "d220" = 6.5
  constraints: 2 centre point, 1 coincident
  measures "d220" diameter of A2
extrude "Extrusion12" cut sketch "Sketch17" against normal blind 75 contours A2
sketch "Sketch18" plane through (-102.0958, 7.69, 6.5001) normal (0, 0, 1) x (1, 0, 0)
  circle A0 centre (33.328, -12) radius 3.25 projected
  circle A1 centre (33.328, -12) radius 5.625
  point P0 (102.0958, -7.69)
  dimension "d223" = 11.25
  constraints: 1 centre point, 1 coincident
  measures "d223" diameter of A1
extrude "Extrusion13" cut sketch "Sketch18" against normal blind 1.2
sketch "Sketch19" plane through (4.0002, 7.69, -59.7999) normal (0, 0, -1) x (-1, 0, 0)
  circle A0 centre (72.768, -12) radius 3.25 projected
  circle A1 centre (72.768, -12) radius 5.625 projected
  point P0 (4.0002, -7.69)
extrude "Extrusion14" cut sketch "Sketch19" against normal blind 1.2
body "Solid1"
